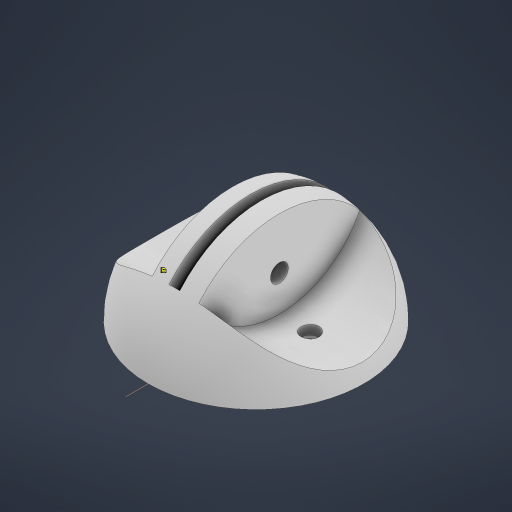
# Autodesk Inventor part: Part1
Saved by Autodesk Inventor 2023 (Build 270158000, 158)
## iProperties
Created: 2022-11-23
Part Number: Part1
Material: Generic
Document SubType Name: Modeling
Designer: iusti
Density: 1 g/cm^3
Appearance: Default
Author: iusti
Autodesk Inventor part; units mm, degrees
ref_plane "XY Plane" through (0, 0, 0) normal (0, 0, 1) x (1, 0, 0)
sketch "Sketch1" plane through (0, 0, 0) normal (1, 0, 0) x (0, 1, 0)
  arc A0 (0, -30) -> (30, 0) centre (0, 0) ccw
  line L0 (30, 0) -> (0, 0)
  line L1 (0, 0) -> (0, -30)
  dimension "d0" = 30
  constraints: 4 end point, 2 point on circle, 1 centre point, 1 coincident, 1 horizontal, 1 vertical
  measures "d0" radius of A0
revolve "Revolution1" add sketch "Sketch1" angle 360 about axis through (0, 30, 0) along (0, -1, 0)
ref_plane "Work Plane1" through (6.5, 0, 0) normal (1, 0, 0) x (0, 1, 0)
sketch "Sketch3" plane through (6.5, 0, 0) normal (1, 0, 0) x (0, 1, 0)
  circle A0 centre (30, 0) radius 25
  line L0 (0, 30) -> (0, -30) projected
  point P0 (0, 0)
  dimension "d7" = 50
  dimension "d8" = 30
  constraints: 1 centre point, 1 horizontal alignment
  measures "d7" diameter of A0
  measures "d8" distance from line of L0 A0.centre
extrude "Extrusion2" cut sketch "Sketch3" along normal through all
mirror "Mirror1" about plane through (0, 0, 0) normal (1, 0, 0) of "Extrusion2"
sketch "Sketch4" plane through (0, 0, 0) normal (1, 0, 0) x (0, 1, 0)
  arc A0 (0, -30) -> (0, 30) centre (0, 0) ccw projected
  circle A1 centre (30, 0) radius 25
  dimension "d11" = 50
  constraints: 1 centre point, 1 horizontal alignment, 1 point on circle
  measures "d11" diameter of A1
extrude "Extrusion3" cut sketch "Sketch4" along normal mid plane 3
sketch "Sketch5" plane through (6.5, 0, 0) normal (1, 0, 0) x (0, 0, -1)
  circle A0 centre (0, 15) radius 2.5
  line L0 (-30, 0) -> (30, 0) projected
  point P0 (0, 0)
  dimension "d14" = 5
  dimension "d15" = 15
  constraints: 1 centre point
  measures "d14" diameter of A0
  measures "d15" distance from line of L0 A0.centre
extrude "Extrusion4" cut sketch "Sketch5" against normal through all
ref_plane "Work Plane2" through (0, 30, 0) normal (0, 1, 0) x (-1, 0, 0)
sketch "Sketch7" plane through (0, 30, 0) normal (0, 1, 0) x (-1, 0, 0)
  line L0 (15, 0) -> (-15, 0) construction
  point P0 (0, 0)
  point P1 (0, 0)
  dimension "d21" = 30
  constraints: 2 end point, 1 coincident, 1 horizontal, 1 midpoint
  measures "d21" distance of L0.start L0.end
hole "Hole1" at (-15, 30, 0) at (15, 30, 0) direction (0, -1, 0) diameter 2.5 end through all counterbore diameter 5 counterbore depth 27.5
body "Solid1"
